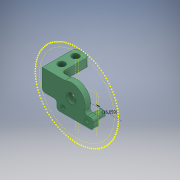
# Autodesk Inventor part: chassis2
Saved by Autodesk Inventor 2019 (Build 230136000, 136)
## iProperties
Created: 2019-09-12
Part Number: chassis2
Material: PET Plastic
Document SubType Name: Modeling
Designer: assman
Density: 1.541 g/cm^3
Appearance: Smooth - Dark Sea Green
Author: assman
## iProperties of the stored document chassis2_3DPrint.ipt
Created: 2019-09-12
Part Number: chassis2_3DPrint
Material: Generic
Document SubType Name: Modeling
Designer: assman
Density: 1 g/cm^3
Appearance: Default
Author: assman
Autodesk Inventor part; units mm, degrees
(part 1 of 2)
ref_plane "YZ Plane" through (0, 0, 0) normal (1, 0, 0) x (0, 1, 0)
ref_plane "XZ Plane" through (0, 0, 0) normal (0, 1, 0) x (-1, 0, 0)
ref_plane "Work Plane2" through (-6.2022, 0, 0) normal (0, 0, 1) x (1, 0, 0)
sketch "Sketch2" plane through (-6.2022, 0, 0) normal (0, 0, 1) x (1, 0, 0)
  circle A0 centre (0, 0) radius 3.35 construction
  circle A1 centre (0, 0) radius 3.35 construction
  line L0 (-6.1, 5.925) -> (-6.1, -5.925) construction
  line L1 (-6.1, -5.925) -> (6.1, -5.925) construction
  line L2 (6.1, -5.925) -> (6.1, 5.925) construction
  line L3 (6.1, 5.925) -> (-6.1, 5.925) construction
  circle A2 centre (0, 0) radius 3.5
  arc A3 (-29.7793, -3.6327) -> (-29.8838, -2.6382) centre (-29.8357, -3.1359) ccw construction
  arc A4 (-29.9286, -2.0692) -> (-29.8838, -2.6382) centre (0, 0) ccw construction
  arc A5 (-29.9286, -2.0692) -> (-29.9809, -1.0706) centre (-29.9589, -1.5701) ccw construction
  arc A6 (-29.9958, -0.5) -> (-29.9809, -1.0706) centre (0, 0) ccw construction
  arc A7 (-29.9958, -0.5) -> (-29.9958, 0.5) centre (-30, 0) ccw construction
  arc A8 (-29.9809, 1.0706) -> (-29.9958, 0.5) centre (0, 0) ccw construction
  arc A9 (-29.9809, 1.0706) -> (-29.9286, 2.0692) centre (-29.9589, 1.5701) ccw construction
  arc A10 (-29.8838, 2.6382) -> (-29.9286, 2.0692) centre (0, 0) ccw construction
  arc A11 (-29.8838, 2.6382) -> (-29.7793, 3.6327) centre (-29.8357, 3.1359) ccw construction
  arc A12 (-29.7047, 4.1986) -> (-29.7793, 3.6327) centre (0, 0) ccw construction
  arc A13 (-29.7047, 4.1986) -> (-29.5483, 5.1862) centre (-29.6307, 4.693) ccw construction
  arc A14 (-29.4443, 5.7474) -> (-29.5483, 5.1862) centre (0, 0) ccw construction
  arc A15 (-29.4443, 5.7474) -> (-29.2364, 6.7255) centre (-29.3444, 6.2374) ccw construction
  arc A16 (-29.1032, 7.2805) -> (-29.2364, 6.7255) centre (0, 0) ccw construction
  arc A17 (-29.1032, 7.2805) -> (-28.8443, 8.2464) centre (-28.9778, 7.7646) ccw construction
  arc A18 (-28.6822, 8.7937) -> (-28.8443, 8.2464) centre (0, 0) ccw construction
  arc A19 (-28.6822, 8.7937) -> (-28.3732, 9.7447) centre (-28.5317, 9.2705) ccw construction
  arc A20 (-28.1827, 10.2828) -> (-28.3732, 9.7447) centre (0, 0) ccw construction
  arc A21 (-28.1827, 10.2828) -> (-27.8243, 11.2163) centre (-28.0074, 10.751) ccw construction
  arc A22 (-27.6059, 11.7436) -> (-27.8243, 11.2163) centre (0, 0) ccw construction
  arc A23 (-27.6059, 11.7436) -> (-27.1992, 12.6572) centre (-27.4064, 12.2021) ccw construction
  arc A24 (-26.9535, 13.1723) -> (-27.1992, 12.6572) centre (0, 0) ccw construction
  arc A25 (-26.9535, 13.1723) -> (-26.4995, 14.0633) centre (-26.7302, 13.6197) ccw construction
  arc A26 (-26.2271, 14.5649) -> (-26.4995, 14.0633) centre (0, 0) ccw construction
  arc A27 (-26.2271, 14.5649) -> (-25.7272, 15.4309) centre (-25.9808, 15) ccw construction
  arc A28 (-25.4289, 15.9176) -> (-25.7272, 15.4309) centre (0, 0) ccw construction
  arc A29 (-25.4289, 15.9176) -> (-24.8843, 16.7562) centre (-25.1601, 16.3392) ccw construction
  arc A30 (-24.561, 17.2266) -> (-24.8843, 16.7562) centre (0, 0) ccw construction
  arc A31 (-24.561, 17.2266) -> (-23.9733, 18.0356) centre (-24.2705, 17.6336) ccw construction
  arc A32 (-23.6258, 18.4884) -> (-23.9733, 18.0356) centre (0, 0) ccw construction
  arc A33 (-23.6258, 18.4884) -> (-22.9965, 19.2655) centre (-23.3144, 18.8796) ccw construction
  arc A34 (-22.6258, 19.6996) -> (-22.9965, 19.2655) centre (0, 0) ccw construction
  arc A35 (-22.6258, 19.6996) -> (-21.9567, 20.4427) centre (-22.2943, 20.0739) ccw construction
  arc A36 (-21.5638, 20.8567) -> (-21.9567, 20.4427) centre (0, 0) ccw construction
  arc A37 (-21.5638, 20.8567) -> (-20.8567, 21.5638) centre (-21.2132, 21.2132) ccw construction
  arc A38 (-20.4427, 21.9567) -> (-20.8567, 21.5638) centre (0, 0) ccw construction
  arc A39 (-20.4427, 21.9567) -> (-19.6996, 22.6258) centre (-20.0739, 22.2943) ccw construction
  arc A40 (-19.2655, 22.9965) -> (-19.6996, 22.6258) centre (0, 0) ccw construction
  arc A41 (-19.2655, 22.9965) -> (-18.4884, 23.6258) centre (-18.8796, 23.3144) ccw construction
  arc A42 (-18.0356, 23.9733) -> (-18.4884, 23.6258) centre (0, 0) ccw construction
  arc A43 (-18.0356, 23.9733) -> (-17.2266, 24.561) centre (-17.6336, 24.2705) ccw construction
  arc A44 (-16.7562, 24.8843) -> (-17.2266, 24.561) centre (0, 0) ccw construction
  arc A45 (-16.7562, 24.8843) -> (-15.9176, 25.4289) centre (-16.3392, 25.1601) ccw construction
  arc A46 (-15.4309, 25.7272) -> (-15.9176, 25.4289) centre (0, 0) ccw construction
  arc A47 (-15.4309, 25.7272) -> (-14.5649, 26.2271) centre (-15, 25.9808) ccw construction
  arc A48 (-14.0633, 26.4995) -> (-14.5649, 26.2271) centre (0, 0) ccw construction
  arc A49 (-14.0633, 26.4995) -> (-13.1723, 26.9535) centre (-13.6197, 26.7302) ccw construction
  arc A50 (-12.6572, 27.1992) -> (-13.1723, 26.9535) centre (0, 0) ccw construction
  arc A51 (-12.6572, 27.1992) -> (-11.7436, 27.6059) centre (-12.2021, 27.4064) ccw construction
  arc A52 (-11.2163, 27.8243) -> (-11.7436, 27.6059) centre (0, 0) ccw construction
  arc A53 (-11.2163, 27.8243) -> (-10.2828, 28.1827) centre (-10.751, 28.0074) ccw construction
  arc A54 (-9.7447, 28.3732) -> (-10.2828, 28.1827) centre (0, 0) ccw construction
  arc A55 (-9.7447, 28.3732) -> (-8.7937, 28.6822) centre (-9.2705, 28.5317) ccw construction
  arc A56 (-8.2464, 28.8443) -> (-8.7937, 28.6822) centre (0, 0) ccw construction
  arc A57 (-8.2464, 28.8443) -> (-7.2805, 29.1032) centre (-7.7646, 28.9778) ccw construction
  arc A58 (-6.7255, 29.2364) -> (-7.2805, 29.1032) centre (0, 0) ccw construction
  arc A59 (-6.7255, 29.2364) -> (-5.7474, 29.4443) centre (-6.2374, 29.3444) ccw construction
  arc A60 (-5.1862, 29.5483) -> (-5.7474, 29.4443) centre (0, 0) ccw construction
  arc A61 (-5.1862, 29.5483) -> (-4.1986, 29.7047) centre (-4.693, 29.6307) ccw construction
  arc A62 (-3.6327, 29.7793) -> (-4.1986, 29.7047) centre (0, 0) ccw construction
  arc A63 (-3.6327, 29.7793) -> (-2.6382, 29.8838) centre (-3.1359, 29.8357) ccw construction
  arc A64 (-2.0692, 29.9286) -> (-2.6382, 29.8838) centre (0, 0) ccw construction
  arc A65 (-2.0692, 29.9286) -> (-1.0706, 29.9809) centre (-1.5701, 29.9589) ccw construction
  arc A66 (-0.5, 29.9958) -> (-1.0706, 29.9809) centre (0, 0) ccw construction
  arc A67 (-0.5, 29.9958) -> (0.5, 29.9958) centre (0, 30) ccw construction
  arc A68 (1.0706, 29.9809) -> (0.5, 29.9958) centre (0, 0) ccw construction
  arc A69 (1.0706, 29.9809) -> (2.0692, 29.9286) centre (1.5701, 29.9589) ccw construction
  arc A70 (2.6382, 29.8838) -> (2.0692, 29.9286) centre (0, 0) ccw construction
  arc A71 (2.6382, 29.8838) -> (3.6327, 29.7793) centre (3.1359, 29.8357) ccw construction
  arc A72 (4.1986, 29.7047) -> (3.6327, 29.7793) centre (0, 0) ccw construction
  arc A73 (4.1986, 29.7047) -> (5.1862, 29.5483) centre (4.693, 29.6307) ccw construction
  arc A74 (5.7474, 29.4443) -> (5.1862, 29.5483) centre (0, 0) ccw construction
  arc A75 (5.7474, 29.4443) -> (6.7255, 29.2364) centre (6.2374, 29.3444) ccw construction
  arc A76 (7.2805, 29.1032) -> (6.7255, 29.2364) centre (0, 0) ccw construction
  arc A77 (7.2805, 29.1032) -> (8.2464, 28.8443) centre (7.7646, 28.9778) ccw construction
  arc A78 (8.7937, 28.6822) -> (8.2464, 28.8443) centre (0, 0) ccw construction
  arc A79 (8.7937, 28.6822) -> (9.7447, 28.3732) centre (9.2705, 28.5317) ccw construction
  arc A80 (10.2828, 28.1827) -> (9.7447, 28.3732) centre (0, 0) ccw construction
  arc A81 (10.2828, 28.1827) -> (11.2163, 27.8243) centre (10.751, 28.0074) ccw construction
  arc A82 (11.7436, 27.6059) -> (11.2163, 27.8243) centre (0, 0) ccw construction
  arc A83 (11.7436, 27.6059) -> (12.6572, 27.1992) centre (12.2021, 27.4064) ccw construction
  arc A84 (13.1723, 26.9535) -> (12.6572, 27.1992) centre (0, 0) ccw construction
  arc A85 (13.1723, 26.9535) -> (14.0633, 26.4995) centre (13.6197, 26.7302) ccw construction
  arc A86 (14.5649, 26.2271) -> (14.0633, 26.4995) centre (0, 0) ccw construction
  arc A87 (14.5649, 26.2271) -> (15.4309, 25.7272) centre (15, 25.9808) ccw construction
  arc A88 (15.9176, 25.4289) -> (15.4309, 25.7272) centre (0, 0) ccw construction
  arc A89 (15.9176, 25.4289) -> (16.7562, 24.8843) centre (16.3392, 25.1601) ccw construction
  arc A90 (17.2266, 24.561) -> (16.7562, 24.8843) centre (0, 0) ccw construction
  arc A91 (17.2266, 24.561) -> (18.0356, 23.9733) centre (17.6336, 24.2705) ccw construction
  arc A92 (18.4884, 23.6258) -> (18.0356, 23.9733) centre (0, 0) ccw construction
  arc A93 (18.4884, 23.6258) -> (19.2655, 22.9965) centre (18.8796, 23.3144) ccw construction
  arc A94 (19.6996, 22.6258) -> (19.2655, 22.9965) centre (0, 0) ccw construction
  arc A95 (19.6996, 22.6258) -> (20.4427, 21.9567) centre (20.0739, 22.2943) ccw construction
  arc A96 (20.8567, 21.5638) -> (20.4427, 21.9567) centre (0, 0) ccw construction
  arc A97 (20.8567, 21.5638) -> (21.5638, 20.8567) centre (21.2132, 21.2132) ccw construction
  arc A98 (21.9567, 20.4427) -> (21.5638, 20.8567) centre (0, 0) ccw construction
  arc A99 (21.9567, 20.4427) -> (22.6258, 19.6996) centre (22.2943, 20.0739) ccw construction
  arc A100 (22.9965, 19.2655) -> (22.6258, 19.6996) centre (0, 0) ccw construction
  arc A101 (22.9965, 19.2655) -> (23.6258, 18.4884) centre (23.3144, 18.8796) ccw construction
  arc A102 (23.9733, 18.0356) -> (23.6258, 18.4884) centre (0, 0) ccw construction
  arc A103 (23.9733, 18.0356) -> (24.561, 17.2266) centre (24.2705, 17.6336) ccw construction
  arc A104 (24.8843, 16.7562) -> (24.561, 17.2266) centre (0, 0) ccw construction
  arc A105 (24.8843, 16.7562) -> (25.4289, 15.9176) centre (25.1601, 16.3392) ccw construction
  arc A106 (25.7272, 15.4309) -> (25.4289, 15.9176) centre (0, 0) ccw construction
  arc A107 (25.7272, 15.4309) -> (26.2271, 14.5649) centre (25.9808, 15) ccw construction
  arc A108 (26.4995, 14.0633) -> (26.2271, 14.5649) centre (0, 0) ccw construction
  arc A109 (26.4995, 14.0633) -> (26.9535, 13.1723) centre (26.7302, 13.6197) ccw construction
  arc A110 (27.1992, 12.6572) -> (26.9535, 13.1723) centre (0, 0) ccw construction
  arc A111 (27.1992, 12.6572) -> (27.6059, 11.7436) centre (27.4064, 12.2021) ccw construction
  arc A112 (27.8243, 11.2163) -> (27.6059, 11.7436) centre (0, 0) ccw construction
  arc A113 (27.8243, 11.2163) -> (28.1827, 10.2828) centre (28.0074, 10.751) ccw construction
  arc A114 (28.3732, 9.7447) -> (28.1827, 10.2828) centre (0, 0) ccw construction
  arc A115 (28.3732, 9.7447) -> (28.6822, 8.7937) centre (28.5317, 9.2705) ccw construction
  arc A116 (28.8443, 8.2464) -> (28.6822, 8.7937) centre (0, 0) ccw construction
  arc A117 (28.8443, 8.2464) -> (29.1032, 7.2805) centre (28.9778, 7.7646) ccw construction
  arc A118 (29.2364, 6.7255) -> (29.1032, 7.2805) centre (0, 0) ccw construction
  arc A119 (29.2364, 6.7255) -> (29.4443, 5.7474) centre (29.3444, 6.2374) ccw construction
  arc A120 (29.5483, 5.1862) -> (29.4443, 5.7474) centre (0, 0) ccw construction
  arc A121 (29.5483, 5.1862) -> (29.7047, 4.1986) centre (29.6307, 4.693) ccw construction
  arc A122 (29.7793, 3.6327) -> (29.7047, 4.1986) centre (0, 0) ccw construction
  arc A123 (29.7793, 3.6327) -> (29.8838, 2.6382) centre (29.8357, 3.1359) ccw construction
  arc A124 (29.9286, 2.0692) -> (29.8838, 2.6382) centre (0, 0) ccw construction
  arc A125 (29.9286, 2.0692) -> (29.9809, 1.0706) centre (29.9589, 1.5701) ccw construction
  arc A126 (29.9958, 0.5) -> (29.9809, 1.0706) centre (0, 0) ccw construction
  arc A127 (29.9958, 0.5) -> (29.9958, -0.5) centre (30, 0) ccw construction
  arc A128 (29.9809, -1.0706) -> (29.9958, -0.5) centre (0, 0) ccw construction
  arc A129 (29.9809, -1.0706) -> (29.9286, -2.0692) centre (29.9589, -1.5701) ccw construction
  arc A130 (29.8838, -2.6382) -> (29.9286, -2.0692) centre (0, 0) ccw construction
  arc A131 (29.8838, -2.6382) -> (29.7793, -3.6327) centre (29.8357, -3.1359) ccw construction
  arc A132 (29.7047, -4.1986) -> (29.7793, -3.6327) centre (0, 0) ccw construction
  arc A133 (29.7047, -4.1986) -> (29.5483, -5.1862) centre (29.6307, -4.693) ccw construction
  arc A134 (29.4443, -5.7474) -> (29.5483, -5.1862) centre (0, 0) ccw construction
  arc A135 (29.4443, -5.7474) -> (29.2364, -6.7255) centre (29.3444, -6.2374) ccw construction
  arc A136 (29.1032, -7.2805) -> (29.2364, -6.7255) centre (0, 0) ccw construction
  arc A137 (29.1032, -7.2805) -> (28.8443, -8.2464) centre (28.9778, -7.7646) ccw construction
  arc A138 (28.6822, -8.7937) -> (28.8443, -8.2464) centre (0, 0) ccw construction
  arc A139 (28.6822, -8.7937) -> (28.3732, -9.7447) centre (28.5317, -9.2705) ccw construction
  arc A140 (28.1827, -10.2828) -> (28.3732, -9.7447) centre (0, 0) ccw construction
  arc A141 (28.1827, -10.2828) -> (27.8243, -11.2163) centre (28.0074, -10.751) ccw construction
  arc A142 (27.6059, -11.7436) -> (27.8243, -11.2163) centre (0, 0) ccw construction
  arc A143 (27.6059, -11.7436) -> (27.1992, -12.6572) centre (27.4064, -12.2021) ccw construction
  arc A144 (26.9535, -13.1723) -> (27.1992, -12.6572) centre (0, 0) ccw construction
  arc A145 (26.9535, -13.1723) -> (26.4995, -14.0633) centre (26.7302, -13.6197) ccw construction
  arc A146 (26.2271, -14.5649) -> (26.4995, -14.0633) centre (0, 0) ccw construction
  arc A147 (26.2271, -14.5649) -> (25.7272, -15.4309) centre (25.9808, -15) ccw construction
  arc A148 (25.4289, -15.9176) -> (25.7272, -15.4309) centre (0, 0) ccw construction
  arc A149 (25.4289, -15.9176) -> (24.8843, -16.7562) centre (25.1601, -16.3392) ccw construction
  arc A150 (24.561, -17.2266) -> (24.8843, -16.7562) centre (0, 0) ccw construction
  arc A151 (24.561, -17.2266) -> (23.9733, -18.0356) centre (24.2705, -17.6336) ccw construction
  arc A152 (23.6258, -18.4884) -> (23.9733, -18.0356) centre (0, 0) ccw construction
  arc A153 (23.6258, -18.4884) -> (22.9965, -19.2655) centre (23.3144, -18.8796) ccw construction
  arc A154 (22.6258, -19.6996) -> (22.9965, -19.2655) centre (0, 0) ccw construction
  arc A155 (22.6258, -19.6996) -> (21.9567, -20.4427) centre (22.2943, -20.0739) ccw construction
  arc A156 (21.5638, -20.8567) -> (21.9567, -20.4427) centre (0, 0) ccw construction
  arc A157 (21.5638, -20.8567) -> (20.8567, -21.5638) centre (21.2132, -21.2132) ccw construction
  arc A158 (20.4427, -21.9567) -> (20.8567, -21.5638) centre (0, 0) ccw construction
  arc A159 (20.4427, -21.9567) -> (19.6996, -22.6258) centre (20.0739, -22.2943) ccw construction
  arc A160 (19.2655, -22.9965) -> (19.6996, -22.6258) centre (0, 0) ccw construction
  arc A161 (19.2655, -22.9965) -> (18.4884, -23.6258) centre (18.8796, -23.3144) ccw construction
  arc A162 (18.0356, -23.9733) -> (18.4884, -23.6258) centre (0, 0) ccw construction
  arc A163 (18.0356, -23.9733) -> (17.2266, -24.561) centre (17.6336, -24.2705) ccw construction
  arc A164 (16.7562, -24.8843) -> (17.2266, -24.561) centre (0, 0) ccw construction
  arc A165 (16.7562, -24.8843) -> (15.9176, -25.4289) centre (16.3392, -25.1601) ccw construction
  arc A166 (15.4309, -25.7272) -> (15.9176, -25.4289) centre (0, 0) ccw construction
  arc A167 (15.4309, -25.7272) -> (14.5649, -26.2271) centre (15, -25.9808) ccw construction
  arc A168 (14.0633, -26.4995) -> (14.5649, -26.2271) centre (0, 0) ccw construction
  arc A169 (14.0633, -26.4995) -> (13.1723, -26.9535) centre (13.6197, -26.7302) ccw construction
  arc A170 (12.6572, -27.1992) -> (13.1723, -26.9535) centre (0, 0) ccw construction
  arc A171 (12.6572, -27.1992) -> (11.7436, -27.6059) centre (12.2021, -27.4064) ccw construction
  arc A172 (11.2163, -27.8243) -> (11.7436, -27.6059) centre (0, 0) ccw construction
  arc A173 (11.2163, -27.8243) -> (10.2828, -28.1827) centre (10.751, -28.0074) ccw construction
  arc A174 (9.7447, -28.3732) -> (10.2828, -28.1827) centre (0, 0) ccw construction
  arc A175 (9.7447, -28.3732) -> (8.7937, -28.6822) centre (9.2705, -28.5317) ccw construction
  arc A176 (8.2464, -28.8443) -> (8.7937, -28.6822) centre (0, 0) ccw construction
  arc A177 (8.2464, -28.8443) -> (7.2805, -29.1032) centre (7.7646, -28.9778) ccw construction
  arc A178 (6.7255, -29.2364) -> (7.2805, -29.1032) centre (0, 0) ccw construction
  arc A179 (6.7255, -29.2364) -> (5.7474, -29.4443) centre (6.2374, -29.3444) ccw construction
  arc A180 (5.1862, -29.5483) -> (5.7474, -29.4443) centre (0, 0) ccw construction
  arc A181 (5.1862, -29.5483) -> (4.1986, -29.7047) centre (4.693, -29.6307) ccw construction
  arc A182 (3.6327, -29.7793) -> (4.1986, -29.7047) centre (0, 0) ccw construction
  arc A183 (3.6327, -29.7793) -> (2.6382, -29.8838) centre (3.1359, -29.8357) ccw construction
  arc A184 (2.0692, -29.9286) -> (2.6382, -29.8838) centre (0, 0) ccw construction
  arc A185 (2.0692, -29.9286) -> (1.0706, -29.9809) centre (1.5701, -29.9589) ccw construction
  arc A186 (0.5, -29.9958) -> (1.0706, -29.9809) centre (0, 0) ccw construction
  arc A187 (0.5, -29.9958) -> (-0.5, -29.9958) centre (0, -30) ccw construction
  arc A188 (-1.0706, -29.9809) -> (-0.5, -29.9958) centre (0, 0) ccw construction
  arc A189 (-1.0706, -29.9809) -> (-2.0692, -29.9286) centre (-1.5701, -29.9589) ccw construction
  arc A190 (-2.6382, -29.8838) -> (-2.0692, -29.9286) centre (0, 0) ccw construction
  arc A191 (-2.6382, -29.8838) -> (-3.6327, -29.7793) centre (-3.1359, -29.8357) ccw construction
  arc A192 (-4.1986, -29.7047) -> (-3.6327, -29.7793) centre (0, 0) ccw construction
  arc A193 (-4.1986, -29.7047) -> (-5.1862, -29.5483) centre (-4.693, -29.6307) ccw construction
  arc A194 (-5.7474, -29.4443) -> (-5.1862, -29.5483) centre (0, 0) ccw construction
  arc A195 (-5.7474, -29.4443) -> (-6.7255, -29.2364) centre (-6.2374, -29.3444) ccw construction
  arc A196 (-7.2805, -29.1032) -> (-6.7255, -29.2364) centre (0, 0) ccw construction
  arc A197 (-7.2805, -29.1032) -> (-8.2464, -28.8443) centre (-7.7646, -28.9778) ccw construction
  arc A198 (-8.7937, -28.6822) -> (-8.2464, -28.8443) centre (0, 0) ccw construction
  arc A199 (-8.7937, -28.6822) -> (-9.7447, -28.3732) centre (-9.2705, -28.5317) ccw construction
  arc A200 (-10.2828, -28.1827) -> (-9.7447, -28.3732) centre (0, 0) ccw construction
  arc A201 (-10.2828, -28.1827) -> (-11.2163, -27.8243) centre (-10.751, -28.0074) ccw construction
  arc A202 (-11.7436, -27.6059) -> (-11.2163, -27.8243) centre (0, 0) ccw construction
  arc A203 (-11.7436, -27.6059) -> (-12.6572, -27.1992) centre (-12.2021, -27.4064) ccw construction
  arc A204 (-13.1723, -26.9535) -> (-12.6572, -27.1992) centre (0, 0) ccw construction
  arc A205 (-13.1723, -26.9535) -> (-14.0633, -26.4995) centre (-13.6197, -26.7302) ccw construction
  arc A206 (-14.5649, -26.2271) -> (-14.0633, -26.4995) centre (0, 0) ccw construction
  arc A207 (-14.5649, -26.2271) -> (-15.4309, -25.7272) centre (-15, -25.9808) ccw construction
  arc A208 (-15.9176, -25.4289) -> (-15.4309, -25.7272) centre (0, 0) ccw construction
  arc A209 (-15.9176, -25.4289) -> (-16.7562, -24.8843) centre (-16.3392, -25.1601) ccw construction
  arc A210 (-17.2266, -24.561) -> (-16.7562, -24.8843) centre (0, 0) ccw construction
  arc A211 (-17.2266, -24.561) -> (-18.0356, -23.9733) centre (-17.6336, -24.2705) ccw construction
  arc A212 (-18.4884, -23.6258) -> (-18.0356, -23.9733) centre (0, 0) ccw construction
  arc A213 (-18.4884, -23.6258) -> (-19.2655, -22.9965) centre (-18.8796, -23.3144) ccw construction
  arc A214 (-19.6996, -22.6258) -> (-19.2655, -22.9965) centre (0, 0) ccw construction
  arc A215 (-19.6996, -22.6258) -> (-20.4427, -21.9567) centre (-20.0739, -22.2943) ccw construction
  arc A216 (-20.8567, -21.5638) -> (-20.4427, -21.9567) centre (0, 0) ccw construction
  arc A217 (-20.8567, -21.5638) -> (-21.5638, -20.8567) centre (-21.2132, -21.2132) ccw construction
  arc A218 (-21.9567, -20.4427) -> (-21.5638, -20.8567) centre (0, 0) ccw construction
  arc A219 (-21.9567, -20.4427) -> (-22.6258, -19.6996) centre (-22.2943, -20.0739) ccw construction
  arc A220 (-22.9965, -19.2655) -> (-22.6258, -19.6996) centre (0, 0) ccw construction
  arc A221 (-22.9965, -19.2655) -> (-23.6258, -18.4884) centre (-23.3144, -18.8796) ccw construction
  arc A222 (-23.9733, -18.0356) -> (-23.6258, -18.4884) centre (0, 0) ccw construction
  arc A223 (-23.9733, -18.0356) -> (-24.561, -17.2266) centre (-24.2705, -17.6336) ccw construction
  arc A224 (-24.8843, -16.7562) -> (-24.561, -17.2266) centre (0, 0) ccw construction
  arc A225 (-24.8843, -16.7562) -> (-25.4289, -15.9176) centre (-25.1601, -16.3392) ccw construction
  arc A226 (-25.7272, -15.4309) -> (-25.4289, -15.9176) centre (0, 0) ccw construction
  arc A227 (-25.7272, -15.4309) -> (-26.2271, -14.5649) centre (-25.9808, -15) ccw construction
  arc A228 (-26.4995, -14.0633) -> (-26.2271, -14.5649) centre (0, 0) ccw construction
  arc A229 (-26.4995, -14.0633) -> (-26.9535, -13.1723) centre (-26.7302, -13.6197) ccw construction
  arc A230 (-27.1992, -12.6572) -> (-26.9535, -13.1723) centre (0, 0) ccw construction
  arc A231 (-27.1992, -12.6572) -> (-27.6059, -11.7436) centre (-27.4064, -12.2021) ccw construction
  arc A232 (-27.8243, -11.2163) -> (-27.6059, -11.7436) centre (0, 0) ccw construction
  arc A233 (-27.8243, -11.2163) -> (-28.1827, -10.2828) centre (-28.0074, -10.751) ccw construction
  arc A234 (-28.3732, -9.7447) -> (-28.1827, -10.2828) centre (0, 0) ccw construction
  arc A235 (-28.3732, -9.7447) -> (-28.6822, -8.7937) centre (-28.5317, -9.2705) ccw construction
  arc A236 (-28.8443, -8.2464) -> (-28.6822, -8.7937) centre (0, 0) ccw construction
  arc A237 (-28.8443, -8.2464) -> (-29.1032, -7.2805) centre (-28.9778, -7.7646) ccw construction
  arc A238 (-29.2364, -6.7255) -> (-29.1032, -7.2805) centre (0, 0) ccw construction
  arc A239 (-29.2364, -6.7255) -> (-29.4443, -5.7474) centre (-29.3444, -6.2374) ccw construction
  arc A240 (-29.5483, -5.1862) -> (-29.4443, -5.7474) centre (0, 0) ccw construction
  arc A241 (-29.5483, -5.1862) -> (-29.7047, -4.1986) centre (-29.6307, -4.693) ccw construction
  arc A242 (-29.7793, -3.6327) -> (-29.7047, -4.1986) centre (0, 0) ccw construction
  circle A243 centre (0, 0) radius 27 construction
  line L4 (-30, 0) -> (0, 0) construction
  line L5 (-13.9945, 14.0151) -> (-13.9945, -11.7918) construction
  line L6 (13.9945, 10) -> (-13.9945, 10)
  line L7 (-13.9945, 10) -> (-13.9945, -10)
  line L8 (-13.9945, -10) -> (13.9945, -10)
  line L9 (13.9945, -10) -> (13.9945, 10)
  point P0 (6.2022, 0)
  dimension "d0" = 7
  dimension "d2" = 16.0055
  dimension "d3" = 20
  constraints: 12 end point, 2 horizontal, 2 parallel, 1 centre point, 1 coincident, 1 perpendicular, 1 point on line, 1 vertical
  measures "d0" diameter of A2
  measures "d2" distance from line of L5 A7.centre
  measures "d3" distance of L7.end L6.end
extrude "Extrusion1" add sketch "Sketch2" along normal blind 2.5
sketch "Sketch3" plane through (-6.2022, 0, 2.5) normal (0, 0, 1) x (-1, 0, 0)
  line L0 (-21.45, -7.175) -> (-11.45, -7.175) projected
  line L1 (-11.45, -7.175) -> (-11.45, 5.225) projected
  line L2 (-11.45, 5.225) -> (-21.45, 5.225) projected
  line L3 (-21.45, 5.225) -> (-21.45, -7.175) projected
  point P0 (-6.2022, 0)
extrude "Extrusion2" cut sketch "Sketch3" against normal blind 1
sketch "Sketch4" plane through (-6.2022, 0, 2.5) normal (0, 0, 1) x (-1, 0, 0)
  circle A0 centre (0, 0) radius 3.35 construction
  line L0 (6.1, -5.925) -> (6.1, 5.925) projected
  line L1 (6.1, 5.925) -> (-6.1, 5.925) projected
  line L2 (-6.1, 5.925) -> (-6.1, -5.925) projected
  line L3 (-6.1, -5.925) -> (6.1, -5.925) projected
  circle A1 centre (5.9, 8.625) radius 1.5 construction
  circle A2 centre (-11.35, 8.625) radius 1.5 construction
  line L4 (10.4, -7.925) -> (-15.85, -7.925) construction
  line L5 (-15.85, -7.925) -> (-15.85, 11.325) construction
  line L6 (-15.85, 11.325) -> (10.4, 11.325) construction
  line L7 (10.4, 11.325) -> (10.4, -7.925) construction
  point P0 (-6.2022, 0)
extrude "Extrusion3" cut sketch "Sketch4" against normal blind 2.5 keep common part
sketch "Sketch5" plane through (-6.2022, 0, 2.5) normal (0, 0, 1) x (1, 0, 0)
  circle A0 centre (0, 0) radius 10
  point P0 (6.2022, 0)
  dimension "d10" = 20
  constraints: 1 centre point
  measures "d10" diameter of A0
extrude "Extrusion4" add sketch "Sketch5" against normal blind 2.5
sketch "Sketch6" plane through (-6.2022, 0, 0) normal (0, 0, -1) x (-1, 0, 0)
  circle A0 centre (0, 0) radius 3.5
  point P0 (-6.2022, 0)
  dimension "d13" = 7
  constraints: 1 centre point
  measures "d13" diameter of A0
extrude "Extrusion5" cut sketch "Sketch6" against normal blind 2.5
sketch "Sketch25" plane through (-6.2022, 0, 0) normal (0, 0, -1) x (-1, 0, 0)
  arc A0 (29.8838, -2.6382) -> (29.7793, -3.6327) centre (29.8357, -3.1359) ccw construction
  arc A1 (29.8838, -2.6382) -> (29.9286, -2.0692) centre (0, 0) ccw construction
  arc A2 (29.9809, -1.0706) -> (29.9286, -2.0692) centre (29.9589, -1.5701) ccw construction
  arc A3 (29.9809, -1.0706) -> (29.9958, -0.5) centre (0, 0) ccw construction
  arc A4 (29.9958, 0.5) -> (29.9958, -0.5) centre (30, 0) ccw construction
  arc A5 (29.9958, 0.5) -> (29.9809, 1.0706) centre (0, 0) ccw construction
  arc A6 (29.9286, 2.0692) -> (29.9809, 1.0706) centre (29.9589, 1.5701) ccw construction
  arc A7 (29.9286, 2.0692) -> (29.8838, 2.6382) centre (0, 0) ccw construction
  arc A8 (29.7793, 3.6327) -> (29.8838, 2.6382) centre (29.8357, 3.1359) ccw construction
  arc A9 (29.7793, 3.6327) -> (29.7047, 4.1986) centre (0, 0) ccw construction
  arc A10 (29.5483, 5.1862) -> (29.7047, 4.1986) centre (29.6307, 4.693) ccw construction
  arc A11 (29.5483, 5.1862) -> (29.4443, 5.7474) centre (0, 0) ccw construction
  arc A12 (29.2364, 6.7255) -> (29.4443, 5.7474) centre (29.3444, 6.2374) ccw construction
  arc A13 (29.2364, 6.7255) -> (29.1032, 7.2805) centre (0, 0) ccw construction
  arc A14 (28.8443, 8.2464) -> (29.1032, 7.2805) centre (28.9778, 7.7646) ccw construction
  arc A15 (28.8443, 8.2464) -> (28.6822, 8.7937) centre (0, 0) ccw construction
  arc A16 (28.3732, 9.7447) -> (28.6822, 8.7937) centre (28.5317, 9.2705) ccw construction
  arc A17 (28.3732, 9.7447) -> (28.1827, 10.2828) centre (0, 0) ccw construction
  arc A18 (27.8243, 11.2163) -> (28.1827, 10.2828) centre (28.0074, 10.751) ccw construction
  arc A19 (27.8243, 11.2163) -> (27.6059, 11.7436) centre (0, 0) ccw construction
  arc A20 (27.1992, 12.6572) -> (27.6059, 11.7436) centre (27.4064, 12.2021) ccw construction
  arc A21 (27.1992, 12.6572) -> (26.9535, 13.1723) centre (0, 0) ccw construction
  arc A22 (26.4995, 14.0633) -> (26.9535, 13.1723) centre (26.7302, 13.6197) ccw construction
  arc A23 (26.4995, 14.0633) -> (26.2271, 14.5649) centre (0, 0) ccw construction
  arc A24 (25.7272, 15.4309) -> (26.2271, 14.5649) centre (25.9808, 15) ccw construction
  arc A25 (25.7272, 15.4309) -> (25.4289, 15.9176) centre (0, 0) ccw construction
  arc A26 (24.8843, 16.7562) -> (25.4289, 15.9176) centre (25.1601, 16.3392) ccw construction
  arc A27 (24.8843, 16.7562) -> (24.561, 17.2266) centre (0, 0) ccw construction
  arc A28 (23.9733, 18.0356) -> (24.561, 17.2266) centre (24.2705, 17.6336) ccw construction
  arc A29 (23.9733, 18.0356) -> (23.6258, 18.4884) centre (0, 0) ccw construction
  arc A30 (22.9965, 19.2655) -> (23.6258, 18.4884) centre (23.3144, 18.8796) ccw construction
  arc A31 (22.9965, 19.2655) -> (22.6258, 19.6996) centre (0, 0) ccw construction
  arc A32 (21.9567, 20.4427) -> (22.6258, 19.6996) centre (22.2943, 20.0739) ccw construction
  arc A33 (21.9567, 20.4427) -> (21.5638, 20.8567) centre (0, 0) ccw construction
  arc A34 (20.8567, 21.5638) -> (21.5638, 20.8567) centre (21.2132, 21.2132) ccw construction
  arc A35 (20.8567, 21.5638) -> (20.4427, 21.9567) centre (0, 0) ccw construction
  arc A36 (19.6996, 22.6258) -> (20.4427, 21.9567) centre (20.0739, 22.2943) ccw construction
  arc A37 (19.6996, 22.6258) -> (19.2655, 22.9965) centre (0, 0) ccw construction
  arc A38 (18.4884, 23.6258) -> (19.2655, 22.9965) centre (18.8796, 23.3144) ccw construction
  arc A39 (18.4884, 23.6258) -> (18.0356, 23.9733) centre (0, 0) ccw construction
  arc A40 (17.2266, 24.561) -> (18.0356, 23.9733) centre (17.6336, 24.2705) ccw construction
  arc A41 (17.2266, 24.561) -> (16.7562, 24.8843) centre (0, 0) ccw construction
  arc A42 (15.9176, 25.4289) -> (16.7562, 24.8843) centre (16.3392, 25.1601) ccw construction
  arc A43 (15.9176, 25.4289) -> (15.4309, 25.7272) centre (0, 0) ccw construction
  arc A44 (14.5649, 26.2271) -> (15.4309, 25.7272) centre (15, 25.9808) ccw construction
  arc A45 (14.5649, 26.2271) -> (14.0633, 26.4995) centre (0, 0) ccw construction
  arc A46 (13.1723, 26.9535) -> (14.0633, 26.4995) centre (13.6197, 26.7302) ccw construction
  arc A47 (13.1723, 26.9535) -> (12.6572, 27.1992) centre (0, 0) ccw construction
  arc A48 (11.7436, 27.6059) -> (12.6572, 27.1992) centre (12.2021, 27.4064) ccw construction
  arc A49 (11.7436, 27.6059) -> (11.2163, 27.8243) centre (0, 0) ccw construction
  arc A50 (10.2828, 28.1827) -> (11.2163, 27.8243) centre (10.751, 28.0074) ccw construction
  arc A51 (10.2828, 28.1827) -> (9.7447, 28.3732) centre (0, 0) ccw construction
  arc A52 (8.7937, 28.6822) -> (9.7447, 28.3732) centre (9.2705, 28.5317) ccw construction
  arc A53 (8.7937, 28.6822) -> (8.2464, 28.8443) centre (0, 0) ccw construction
  arc A54 (7.2805, 29.1032) -> (8.2464, 28.8443) centre (7.7646, 28.9778) ccw construction
  arc A55 (7.2805, 29.1032) -> (6.7255, 29.2364) centre (0, 0) ccw construction
  arc A56 (5.7474, 29.4443) -> (6.7255, 29.2364) centre (6.2374, 29.3444) ccw construction
  arc A57 (5.7474, 29.4443) -> (5.1862, 29.5483) centre (0, 0) ccw construction
  arc A58 (4.1986, 29.7047) -> (5.1862, 29.5483) centre (4.693, 29.6307) ccw construction
  arc A59 (4.1986, 29.7047) -> (3.6327, 29.7793) centre (0, 0) ccw construction
  arc A60 (2.6382, 29.8838) -> (3.6327, 29.7793) centre (3.1359, 29.8357) ccw construction
  arc A61 (2.6382, 29.8838) -> (2.0692, 29.9286) centre (0, 0) ccw construction
  arc A62 (1.0706, 29.9809) -> (2.0692, 29.9286) centre (1.5701, 29.9589) ccw construction
  arc A63 (1.0706, 29.9809) -> (0.5, 29.9958) centre (0, 0) ccw construction
  arc A64 (-0.5, 29.9958) -> (0.5, 29.9958) centre (0, 30) ccw construction
  arc A65 (-0.5, 29.9958) -> (-1.0706, 29.9809) centre (0, 0) ccw construction
  arc A66 (-2.0692, 29.9286) -> (-1.0706, 29.9809) centre (-1.5701, 29.9589) ccw construction
  arc A67 (-2.0692, 29.9286) -> (-2.6382, 29.8838) centre (0, 0) ccw construction
  arc A68 (-3.6327, 29.7793) -> (-2.6382, 29.8838) centre (-3.1359, 29.8357) ccw construction
  arc A69 (-3.6327, 29.7793) -> (-4.1986, 29.7047) centre (0, 0) ccw construction
  arc A70 (-5.1862, 29.5483) -> (-4.1986, 29.7047) centre (-4.693, 29.6307) ccw construction
  arc A71 (-5.1862, 29.5483) -> (-5.7474, 29.4443) centre (0, 0) ccw construction
  arc A72 (-6.7255, 29.2364) -> (-5.7474, 29.4443) centre (-6.2374, 29.3444) ccw construction
  arc A73 (-6.7255, 29.2364) -> (-7.2805, 29.1032) centre (0, 0) ccw construction
  arc A74 (-8.2464, 28.8443) -> (-7.2805, 29.1032) centre (-7.7646, 28.9778) ccw construction
  arc A75 (-8.2464, 28.8443) -> (-8.7937, 28.6822) centre (0, 0) ccw construction
  arc A76 (-9.7447, 28.3732) -> (-8.7937, 28.6822) centre (-9.2705, 28.5317) ccw construction
  arc A77 (-9.7447, 28.3732) -> (-10.2828, 28.1827) centre (0, 0) ccw construction
  arc A78 (-11.2163, 27.8243) -> (-10.2828, 28.1827) centre (-10.751, 28.0074) ccw construction
  arc A79 (-11.2163, 27.8243) -> (-11.7436, 27.6059) centre (0, 0) ccw construction
  arc A80 (-12.6572, 27.1992) -> (-11.7436, 27.6059) centre (-12.2021, 27.4064) ccw construction
  arc A81 (-12.6572, 27.1992) -> (-13.1723, 26.9535) centre (0, 0) ccw construction
  arc A82 (-14.0633, 26.4995) -> (-13.1723, 26.9535) centre (-13.6197, 26.7302) ccw construction
  arc A83 (-14.0633, 26.4995) -> (-14.5649, 26.2271) centre (0, 0) ccw construction
  arc A84 (-15.4309, 25.7272) -> (-14.5649, 26.2271) centre (-15, 25.9808) ccw construction
  arc A85 (-15.4309, 25.7272) -> (-15.9176, 25.4289) centre (0, 0) ccw construction
  arc A86 (-16.7562, 24.8843) -> (-15.9176, 25.4289) centre (-16.3392, 25.1601) ccw construction
  arc A87 (-16.7562, 24.8843) -> (-17.2266, 24.561) centre (0, 0) ccw construction
  arc A88 (-18.0356, 23.9733) -> (-17.2266, 24.561) centre (-17.6336, 24.2705) ccw construction
  arc A89 (-18.0356, 23.9733) -> (-18.4884, 23.6258) centre (0, 0) ccw construction
  arc A90 (-19.2655, 22.9965) -> (-18.4884, 23.6258) centre (-18.8796, 23.3144) ccw construction
  arc A91 (-19.2655, 22.9965) -> (-19.6996, 22.6258) centre (0, 0) ccw construction
  arc A92 (-20.4427, 21.9567) -> (-19.6996, 22.6258) centre (-20.0739, 22.2943) ccw construction
  arc A93 (-20.4427, 21.9567) -> (-20.8567, 21.5638) centre (0, 0) ccw construction
  arc A94 (-21.5638, 20.8567) -> (-20.8567, 21.5638) centre (-21.2132, 21.2132) ccw construction
  arc A95 (-21.5638, 20.8567) -> (-21.9567, 20.4427) centre (0, 0) ccw construction
  arc A96 (-22.6258, 19.6996) -> (-21.9567, 20.4427) centre (-22.2943, 20.0739) ccw construction
  arc A97 (-22.6258, 19.6996) -> (-22.9965, 19.2655) centre (0, 0) ccw construction
  arc A98 (-23.6258, 18.4884) -> (-22.9965, 19.2655) centre (-23.3144, 18.8796) ccw construction
  arc A99 (-23.6258, 18.4884) -> (-23.9733, 18.0356) centre (0, 0) ccw construction
  arc A100 (-24.561, 17.2266) -> (-23.9733, 18.0356) centre (-24.2705, 17.6336) ccw construction
  arc A101 (-24.561, 17.2266) -> (-24.8843, 16.7562) centre (0, 0) ccw construction
  arc A102 (-25.4289, 15.9176) -> (-24.8843, 16.7562) centre (-25.1601, 16.3392) ccw construction
  arc A103 (-25.4289, 15.9176) -> (-25.7272, 15.4309) centre (0, 0) ccw construction
  arc A104 (-26.2271, 14.5649) -> (-25.7272, 15.4309) centre (-25.9808, 15) ccw construction
  arc A105 (-26.2271, 14.5649) -> (-26.4995, 14.0633) centre (0, 0) ccw construction
  arc A106 (-26.9535, 13.1723) -> (-26.4995, 14.0633) centre (-26.7302, 13.6197) ccw construction
  arc A107 (-26.9535, 13.1723) -> (-27.1992, 12.6572) centre (0, 0) ccw construction
  arc A108 (-27.6059, 11.7436) -> (-27.1992, 12.6572) centre (-27.4064, 12.2021) ccw construction
  arc A109 (-27.6059, 11.7436) -> (-27.8243, 11.2163) centre (0, 0) ccw construction
  arc A110 (-28.1827, 10.2828) -> (-27.8243, 11.2163) centre (-28.0074, 10.751) ccw construction
  arc A111 (-28.1827, 10.2828) -> (-28.3732, 9.7447) centre (0, 0) ccw construction
  arc A112 (-28.6822, 8.7937) -> (-28.3732, 9.7447) centre (-28.5317, 9.2705) ccw construction
  arc A113 (-28.6822, 8.7937) -> (-28.8443, 8.2464) centre (0, 0) ccw construction
  arc A114 (-29.1032, 7.2805) -> (-28.8443, 8.2464) centre (-28.9778, 7.7646) ccw construction
  arc A115 (-29.1032, 7.2805) -> (-29.2364, 6.7255) centre (0, 0) ccw construction
  arc A116 (-29.4443, 5.7474) -> (-29.2364, 6.7255) centre (-29.3444, 6.2374) ccw construction
  arc A117 (-29.4443, 5.7474) -> (-29.5483, 5.1862) centre (0, 0) ccw construction
  arc A118 (-29.7047, 4.1986) -> (-29.5483, 5.1862) centre (-29.6307, 4.693) ccw construction
  arc A119 (-29.7047, 4.1986) -> (-29.7793, 3.6327) centre (0, 0) ccw construction
  arc A120 (-29.8838, 2.6382) -> (-29.7793, 3.6327) centre (-29.8357, 3.1359) ccw construction
  arc A121 (-29.8838, 2.6382) -> (-29.9286, 2.0692) centre (0, 0) ccw construction
  arc A122 (-29.9809, 1.0706) -> (-29.9286, 2.0692) centre (-29.9589, 1.5701) ccw construction
  arc A123 (-29.9809, 1.0706) -> (-29.9958, 0.5) centre (0, 0) ccw construction
  arc A124 (-29.9958, -0.5) -> (-29.9958, 0.5) centre (-30, 0) ccw construction
  arc A125 (-29.9958, -0.5) -> (-29.9809, -1.0706) centre (0, 0) ccw construction
  arc A126 (-29.9286, -2.0692) -> (-29.9809, -1.0706) centre (-29.9589, -1.5701) ccw construction
  arc A127 (-29.9286, -2.0692) -> (-29.8838, -2.6382) centre (0, 0) ccw construction
  arc A128 (-29.7793, -3.6327) -> (-29.8838, -2.6382) centre (-29.8357, -3.1359) ccw construction
  arc A129 (-29.7793, -3.6327) -> (-29.7047, -4.1986) centre (0, 0) ccw construction
  arc A130 (-29.5483, -5.1862) -> (-29.7047, -4.1986) centre (-29.6307, -4.693) ccw construction
  arc A131 (-29.5483, -5.1862) -> (-29.4443, -5.7474) centre (0, 0) ccw construction
  arc A132 (-29.2364, -6.7255) -> (-29.4443, -5.7474) centre (-29.3444, -6.2374) ccw construction
  arc A133 (-29.2364, -6.7255) -> (-29.1032, -7.2805) centre (0, 0) ccw construction
  arc A134 (-28.8443, -8.2464) -> (-29.1032, -7.2805) centre (-28.9778, -7.7646) ccw construction
  arc A135 (-28.8443, -8.2464) -> (-28.6822, -8.7937) centre (0, 0) ccw construction
  arc A136 (-28.3732, -9.7447) -> (-28.6822, -8.7937) centre (-28.5317, -9.2705) ccw construction
  arc A137 (-28.3732, -9.7447) -> (-28.1827, -10.2828) centre (0, 0) ccw construction
  arc A138 (-27.8243, -11.2163) -> (-28.1827, -10.2828) centre (-28.0074, -10.751) ccw construction
  arc A139 (-27.8243, -11.2163) -> (-27.6059, -11.7436) centre (0, 0) ccw construction
  arc A140 (-27.1992, -12.6572) -> (-27.6059, -11.7436) centre (-27.4064, -12.2021) ccw construction
  arc A141 (-27.1992, -12.6572) -> (-26.9535, -13.1723) centre (0, 0) ccw construction
  arc A142 (-26.4995, -14.0633) -> (-26.9535, -13.1723) centre (-26.7302, -13.6197) ccw construction
  arc A143 (-26.4995, -14.0633) -> (-26.2271, -14.5649) centre (0, 0) ccw construction
  arc A144 (-25.7272, -15.4309) -> (-26.2271, -14.5649) centre (-25.9808, -15) ccw construction
  arc A145 (-25.7272, -15.4309) -> (-25.4289, -15.9176) centre (0, 0) ccw construction
  arc A146 (-24.8843, -16.7562) -> (-25.4289, -15.9176) centre (-25.1601, -16.3392) ccw construction
  arc A147 (-24.8843, -16.7562) -> (-24.561, -17.2266) centre (0, 0) ccw construction
  arc A148 (-23.9733, -18.0356) -> (-24.561, -17.2266) centre (-24.2705, -17.6336) ccw construction
  arc A149 (-23.9733, -18.0356) -> (-23.6258, -18.4884) centre (0, 0) ccw construction
  arc A150 (-22.9965, -19.2655) -> (-23.6258, -18.4884) centre (-23.3144, -18.8796) ccw construction
  arc A151 (-22.9965, -19.2655) -> (-22.6258, -19.6996) centre (0, 0) ccw construction
  arc A152 (-21.9567, -20.4427) -> (-22.6258, -19.6996) centre (-22.2943, -20.0739) ccw construction
  arc A153 (-21.9567, -20.4427) -> (-21.5638, -20.8567) centre (0, 0) ccw construction
  arc A154 (-20.8567, -21.5638) -> (-21.5638, -20.8567) centre (-21.2132, -21.2132) ccw construction
  arc A155 (-20.8567, -21.5638) -> (-20.4427, -21.9567) centre (0, 0) ccw construction
  arc A156 (-19.6996, -22.6258) -> (-20.4427, -21.9567) centre (-20.0739, -22.2943) ccw construction
  arc A157 (-19.6996, -22.6258) -> (-19.2655, -22.9965) centre (0, 0) ccw construction
  arc A158 (-18.4884, -23.6258) -> (-19.2655, -22.9965) centre (-18.8796, -23.3144) ccw construction
  arc A159 (-18.4884, -23.6258) -> (-18.0356, -23.9733) centre (0, 0) ccw construction
  arc A160 (-17.2266, -24.561) -> (-18.0356, -23.9733) centre (-17.6336, -24.2705) ccw construction
  arc A161 (-17.2266, -24.561) -> (-16.7562, -24.8843) centre (0, 0) ccw construction
  arc A162 (-15.9176, -25.4289) -> (-16.7562, -24.8843) centre (-16.3392, -25.1601) ccw construction
  arc A163 (-15.9176, -25.4289) -> (-15.4309, -25.7272) centre (0, 0) ccw construction
  arc A164 (-14.5649, -26.2271) -> (-15.4309, -25.7272) centre (-15, -25.9808) ccw construction
  arc A165 (-14.5649, -26.2271) -> (-14.0633, -26.4995) centre (0, 0) ccw construction
  arc A166 (-13.1723, -26.9535) -> (-14.0633, -26.4995) centre (-13.6197, -26.7302) ccw construction
  arc A167 (-13.1723, -26.9535) -> (-12.6572, -27.1992) centre (0, 0) ccw construction
  arc A168 (-11.7436, -27.6059) -> (-12.6572, -27.1992) centre (-12.2021, -27.4064) ccw construction
  arc A169 (-11.7436, -27.6059) -> (-11.2163, -27.8243) centre (0, 0) ccw construction
  arc A170 (-10.2828, -28.1827) -> (-11.2163, -27.8243) centre (-10.751, -28.0074) ccw construction
  arc A171 (-10.2828, -28.1827) -> (-9.7447, -28.3732) centre (0, 0) ccw construction
  arc A172 (-8.7937, -28.6822) -> (-9.7447, -28.3732) centre (-9.2705, -28.5317) ccw construction
  arc A173 (-8.7937, -28.6822) -> (-8.2464, -28.8443) centre (0, 0) ccw construction
  arc A174 (-7.2805, -29.1032) -> (-8.2464, -28.8443) centre (-7.7646, -28.9778) ccw construction
  arc A175 (-7.2805, -29.1032) -> (-6.7255, -29.2364) centre (0, 0) ccw construction
  arc A176 (-5.7474, -29.4443) -> (-6.7255, -29.2364) centre (-6.2374, -29.3444) ccw construction
  arc A177 (-5.7474, -29.4443) -> (-5.1862, -29.5483) centre (0, 0) ccw construction
  arc A178 (-4.1986, -29.7047) -> (-5.1862, -29.5483) centre (-4.693, -29.6307) ccw construction
  arc A179 (-4.1986, -29.7047) -> (-3.6327, -29.7793) centre (0, 0) ccw construction
  arc A180 (-2.6382, -29.8838) -> (-3.6327, -29.7793) centre (-3.1359, -29.8357) ccw construction
  arc A181 (-2.6382, -29.8838) -> (-2.0692, -29.9286) centre (0, 0) ccw construction
  arc A182 (-1.0706, -29.9809) -> (-2.0692, -29.9286) centre (-1.5701, -29.9589) ccw construction
  arc A183 (-1.0706, -29.9809) -> (-0.5, -29.9958) centre (0, 0) ccw construction
  arc A184 (0.5, -29.9958) -> (-0.5, -29.9958) centre (0, -30) ccw construction
  arc A185 (0.5, -29.9958) -> (1.0706, -29.9809) centre (0, 0) ccw construction
  arc A186 (2.0692, -29.9286) -> (1.0706, -29.9809) centre (1.5701, -29.9589) ccw construction
  arc A187 (2.0692, -29.9286) -> (2.6382, -29.8838) centre (0, 0) ccw construction
  arc A188 (3.6327, -29.7793) -> (2.6382, -29.8838) centre (3.1359, -29.8357) ccw construction
  arc A189 (3.6327, -29.7793) -> (4.1986, -29.7047) centre (0, 0) ccw construction
  arc A190 (5.1862, -29.5483) -> (4.1986, -29.7047) centre (4.693, -29.6307) ccw construction
  arc A191 (5.1862, -29.5483) -> (5.7474, -29.4443) centre (0, 0) ccw construction
  arc A192 (6.7255, -29.2364) -> (5.7474, -29.4443) centre (6.2374, -29.3444) ccw construction
  arc A193 (6.7255, -29.2364) -> (7.2805, -29.1032) centre (0, 0) ccw construction
  arc A194 (8.2464, -28.8443) -> (7.2805, -29.1032) centre (7.7646, -28.9778) ccw construction
  arc A195 (8.2464, -28.8443) -> (8.7937, -28.6822) centre (0, 0) ccw construction
  arc A196 (9.7447, -28.3732) -> (8.7937, -28.6822) centre (9.2705, -28.5317) ccw construction
  arc A197 (9.7447, -28.3732) -> (10.2828, -28.1827) centre (0, 0) ccw construction
  arc A198 (11.2163, -27.8243) -> (10.2828, -28.1827) centre (10.751, -28.0074) ccw construction
  arc A199 (11.2163, -27.8243) -> (11.7436, -27.6059) centre (0, 0) ccw construction
  arc A200 (12.6572, -27.1992) -> (11.7436, -27.6059) centre (12.2021, -27.4064) ccw construction
  arc A201 (12.6572, -27.1992) -> (13.1723, -26.9535) centre (0, 0) ccw construction
  arc A202 (14.0633, -26.4995) -> (13.1723, -26.9535) centre (13.6197, -26.7302) ccw construction
  arc A203 (14.0633, -26.4995) -> (14.5649, -26.2271) centre (0, 0) ccw construction
  arc A204 (15.4309, -25.7272) -> (14.5649, -26.2271) centre (15, -25.9808) ccw construction
  arc A205 (15.4309, -25.7272) -> (15.9176, -25.4289) centre (0, 0) ccw construction
  arc A206 (16.7562, -24.8843) -> (15.9176, -25.4289) centre (16.3392, -25.1601) ccw construction
  arc A207 (16.7562, -24.8843) -> (17.2266, -24.561) centre (0, 0) ccw construction
  arc A208 (18.0356, -23.9733) -> (17.2266, -24.561) centre (17.6336, -24.2705) ccw construction
  arc A209 (18.0356, -23.9733) -> (18.4884, -23.6258) centre (0, 0) ccw construction
  arc A210 (19.2655, -22.9965) -> (18.4884, -23.6258) centre (18.8796, -23.3144) ccw construction
  arc A211 (19.2655, -22.9965) -> (19.6996, -22.6258) centre (0, 0) ccw construction
  arc A212 (20.4427, -21.9567) -> (19.6996, -22.6258) centre (20.0739, -22.2943) ccw construction
  arc A213 (20.4427, -21.9567) -> (20.8567, -21.5638) centre (0, 0) ccw construction
  arc A214 (21.5638, -20.8567) -> (20.8567, -21.5638) centre (21.2132, -21.2132) ccw construction
  arc A215 (21.5638, -20.8567) -> (21.9567, -20.4427) centre (0, 0) ccw construction
  arc A216 (22.6258, -19.6996) -> (21.9567, -20.4427) centre (22.2943, -20.0739) ccw construction
  arc A217 (22.6258, -19.6996) -> (22.9965, -19.2655) centre (0, 0) ccw construction
  arc A218 (23.6258, -18.4884) -> (22.9965, -19.2655) centre (23.3144, -18.8796) ccw construction
  arc A219 (23.6258, -18.4884) -> (23.9733, -18.0356) centre (0, 0) ccw construction
  arc A220 (24.561, -17.2266) -> (23.9733, -18.0356) centre (24.2705, -17.6336) ccw construction
  arc A221 (24.561, -17.2266) -> (24.8843, -16.7562) centre (0, 0) ccw construction
  arc A222 (25.4289, -15.9176) -> (24.8843, -16.7562) centre (25.1601, -16.3392) ccw construction
  arc A223 (25.4289, -15.9176) -> (25.7272, -15.4309) centre (0, 0) ccw construction
  arc A224 (26.2271, -14.5649) -> (25.7272, -15.4309) centre (25.9808, -15) ccw construction
  arc A225 (26.2271, -14.5649) -> (26.4995, -14.0633) centre (0, 0) ccw construction
  arc A226 (26.9535, -13.1723) -> (26.4995, -14.0633) centre (26.7302, -13.6197) ccw construction
  arc A227 (26.9535, -13.1723) -> (27.1992, -12.6572) centre (0, 0) ccw construction
  arc A228 (27.6059, -11.7436) -> (27.1992, -12.6572) centre (27.4064, -12.2021) ccw construction
  arc A229 (27.6059, -11.7436) -> (27.8243, -11.2163) centre (0, 0) ccw construction
  arc A230 (28.1827, -10.2828) -> (27.8243, -11.2163) centre (28.0074, -10.751) ccw construction
  arc A231 (28.1827, -10.2828) -> (28.3732, -9.7447) centre (0, 0) ccw construction
  arc A232 (28.6822, -8.7937) -> (28.3732, -9.7447) centre (28.5317, -9.2705) ccw construction
  arc A233 (28.6822, -8.7937) -> (28.8443, -8.2464) centre (0, 0) ccw construction
  arc A234 (29.1032, -7.2805) -> (28.8443, -8.2464) centre (28.9778, -7.7646) ccw construction
  arc A235 (29.1032, -7.2805) -> (29.2364, -6.7255) centre (0, 0) ccw construction
  arc A236 (29.4443, -5.7474) -> (29.2364, -6.7255) centre (29.3444, -6.2374) ccw construction
  arc A237 (29.4443, -5.7474) -> (29.5483, -5.1862) centre (0, 0) ccw construction
  arc A238 (29.7047, -4.1986) -> (29.5483, -5.1862) centre (29.6307, -4.693) ccw construction
  arc A239 (29.7047, -4.1986) -> (29.7793, -3.6327) centre (0, 0) ccw construction
  circle A240 centre (0, 0) radius 27 construction
  line L0 (1, 13.0767) -> (1, 22.8035) construction
  line L1 (-1, 22.8035) -> (-1, 13.0767) construction
  arc A241 (1.0076, 22.9779) -> (-1.0076, 22.9779) centre (0, 0) ccw construction
  line L2 (-1, -13.0767) -> (-1, -22.8035) construction
  line L3 (1, -22.8035) -> (1, -13.0767) construction
  arc A242 (-1.0076, -22.9779) -> (1.0076, -22.9779) centre (0, 0) ccw construction
  circle A243 centre (5.9, -8.625) radius 1.5 construction
  circle A244 centre (-11.35, -8.625) radius 1.5 construction
  line L4 (10.4, 7.925) -> (-15.85, 7.925) construction
  line L5 (-15.85, 7.925) -> (-15.85, -11.325) construction
  line L6 (-15.85, -11.325) -> (10.4, -11.325) construction
  line L7 (10.4, -11.325) -> (10.4, 7.925) construction
  line L8 (0, 0) -> (-32.9792, 0) construction
  line L9 (-13.9407, 9.2916) -> (-13.9407, -18.7912) construction
  line L10 (0, 11.2163) -> (0, -11.325) construction
  point P0 (-6.2022, 0)
  point P1 (19.2655, 0)
  dimension "d102" = 16.0592
  constraints: 6 end point, 2 point on line, 1 horizontal, 1 perpendicular, 1 vertical
  measures "d102" distance from line of A124.centre L9
thicken "Thicken12" operation add thickness 1.5 both sides no extend neighbours yes toward (0, 0, 1) faces at (1.5004, -1.0769, 2.5)
sketch "Sketch39" plane through (-6.2022, 0, 0) normal (0, 0, -1) x (-1, 0, 0)
  circle A0 centre (0, 0) radius 3.5 projected
  circle A1 centre (0, 0) radius 10 projected
  circle A2 centre (0, 0) radius 10 projected
  line L0 (4.4538, 8.9534) -> (16.4538, 8.9534)
  line L1 (16.4538, 8.9534) -> (16.4538, -6.0466)
  line L2 (16.4538, -6.0466) -> (7.9648, -6.0466)
  point P0 (-6.2022, 0)
  dimension "d189" = 12
  dimension "d190" = 15
  constraints: 6 end point, 2 point on circle, 1 perpendicular, 1 vertical
  measures "d189" distance of L0.start L0.end
  measures "d190" distance of L0.end L1.end
extrude "Extrusion29" add sketch "Sketch39" against normal blind 4 contours A1 L0 L1 L2
thicken "Thicken13" operation add thickness 1.5 both sides no extend neighbours yes toward (-1, 0, 0) faces at (-22.656, -1.0466, 1.3333)
thicken "Thicken14" operation add thickness 1 both sides no extend neighbours yes toward (-1, 0, 0) faces at (-24.156, -1.0466, 1.3333)
thicken "Thicken15" operation add thickness 1 both sides no extend neighbours yes toward (-1, 0, 0) faces at (-25.156, -1.0466, 1.3333)
thicken "Thicken16" operation add thickness 1 both sides no extend neighbours yes toward (-1, 0, 0) faces at (-26.156, -1.0466, 1.3333)